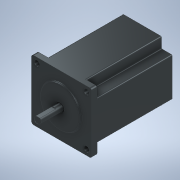
# Autodesk Inventor part: 0x002
Saved by Autodesk Inventor 2020 (Build 240168000, 168)
## iProperties
Created: 2024-01-28
Part Number: 0x002
Material: Iron, Cast
Document SubType Name: Modeling
Designer: Scott Bricker
Density: 7.15 g/cm^3
Appearance: Iron Gray
Mass: 1598.08 g
Surface Area: 245.33 cm^2
Volume: 223.508 cm^3
Project: Motorized Rotator Mount
Description: Stepper Motor
Engineer: Scott Bricker
Author: Scott Bricker
Title: Stepper Motor
Comments: Re-modeled replica of StepperOnline NEMA23 stepper motor for modeling purposes.
Revision Number: v1.0
Autodesk Inventor part; units mm, degrees
ref_plane "YZ Plane" through (0, 0, 0) normal (1, 0, 0) x (0, 1, 0)
ref_plane "XZ Plane" through (0, 0, 0) normal (0, 1, 0) x (-1, 0, 0)
ref_plane "XY Plane" through (0, 0, 0) normal (0, 0, 1) x (1, 0, 0)
sketch "Sketch1" plane through (0, 0, 0) normal (0, 0, 1) x (1, 0, 0)
  line L0 (11.16, 0) -> (46.14, 0)
  line L1 (57.3, 11.16) -> (57.3, 46.14)
  line L2 (46.14, 57.3) -> (11.16, 57.3)
  line L3 (0, 46.14) -> (0, 11.16)
  line L4 (0, 0) -> (0, 10.16)
  line L5 (1, 10.16) -> (9.16, 10.16)
  line L6 (10.16, 9.16) -> (10.16, 1)
  line L7 (57.3, 0) -> (47.14, 0)
  line L8 (47.14, 1) -> (47.14, 9.16)
  line L9 (48.14, 10.16) -> (56.3, 10.16)
  line L10 (47.14, 56.3) -> (47.14, 48.14)
  line L11 (48.14, 47.14) -> (56.3, 47.14)
  line L12 (10.16, 56.3) -> (10.16, 48.14)
  line L13 (1, 47.14) -> (9.16, 47.14)
  arc A0 (9.16, 47.14) -> (10.16, 48.14) centre (9.16, 48.14) ccw
  arc A1 (47.14, 48.14) -> (48.14, 47.14) centre (48.14, 48.14) ccw
  arc A2 (10.16, 9.16) -> (9.16, 10.16) centre (9.16, 9.16) ccw
  arc A3 (48.14, 10.16) -> (47.14, 9.16) centre (48.14, 9.16) ccw
  arc A4 (11.16, 57.3) -> (10.16, 56.3) centre (11.16, 56.3) ccw
  arc A5 (47.14, 56.3) -> (46.14, 57.3) centre (46.14, 56.3) ccw
  arc A6 (57.3, 46.14) -> (56.3, 47.14) centre (56.3, 46.14) ccw
  arc A7 (56.3, 10.16) -> (57.3, 11.16) centre (56.3, 11.16) ccw
  arc A8 (46.14, 0) -> (47.14, 1) centre (46.14, 1) ccw
  arc A9 (10.16, 1) -> (11.16, 0) centre (11.16, 1) ccw
  arc A10 (0, 11.16) -> (1, 10.16) centre (1, 11.16) ccw
  arc A11 (1, 47.14) -> (0, 46.14) centre (1, 46.14) ccw
  point P0 (57.3, 57.3)
  point P1 (0, 47.14)
  point P2 (10.16, 10.16)
  point P3 (47.14, 10.16)
  point P4 (47.14, 47.14)
  point P5 (10.16, 47.14)
  point P6 (10.16, 57.3)
  point P7 (47.14, 57.3)
  point P8 (57.3, 10.16)
  dimension "d25" = 57.3
  dimension "d26" = 57.3
  dimension "d27" = 10.16
  dimension "d28" = 10.16
  dimension "d29" = 10.16
  dimension "d30" = 10.16
  dimension "d31" = 1
  constraints: 31 point on line, 28 end point, 24 point on circle, 24 tangent, 12 centre point, 11 equal radius, 8 perpendicular, 1 horizontal
  measures "d25" distance of L4.start L7.start
  measures "d26" distance of L7.start point (57.3, 57.3)
  measures "d27" distance of L4.start L4.end
  measures "d28" distance of L4.end point (10.16, 10.16)
  measures "d29" distance of L7.start L7.end
  measures "d30" distance of point (47.14, 57.3) point (47.14, 47.14)
  measures "d31" radius of A0
extrude "Extrusion4" add sketch "Sketch1" along normal blind 76.5
sketch "Sketch4" plane through (0, 0, 76.5) normal (0, 0, 1) x (1, 0, 0)
  arc A0 (10.16, 1) -> (11.16, 0) centre (11.16, 1) ccw projected
  line L0 (11.16, 0) -> (46.14, 0) projected
  arc A1 (46.14, 0) -> (47.14, 1) centre (46.14, 1) ccw projected
  line L1 (47.14, 1) -> (47.14, 9.16) projected
  arc A2 (48.14, 10.16) -> (47.14, 9.16) centre (48.14, 9.16) ccw projected
  line L2 (48.14, 10.16) -> (56.3, 10.16) projected
  arc A3 (56.3, 10.16) -> (57.3, 11.16) centre (56.3, 11.16) ccw projected
  line L3 (57.3, 11.16) -> (57.3, 46.14) projected
  arc A4 (57.3, 46.14) -> (56.3, 47.14) centre (56.3, 46.14) ccw projected
  line L4 (56.3, 47.14) -> (48.14, 47.14) projected
  arc A5 (47.14, 48.14) -> (48.14, 47.14) centre (48.14, 48.14) ccw projected
  line L5 (47.14, 48.14) -> (47.14, 56.3) projected
  arc A6 (47.14, 56.3) -> (46.14, 57.3) centre (46.14, 56.3) ccw projected
  line L6 (46.14, 57.3) -> (11.16, 57.3) projected
  arc A7 (11.16, 57.3) -> (10.16, 56.3) centre (11.16, 56.3) ccw projected
  line L7 (10.16, 56.3) -> (10.16, 48.14) projected
  arc A8 (9.16, 47.14) -> (10.16, 48.14) centre (9.16, 48.14) ccw projected
  line L8 (9.16, 47.14) -> (1, 47.14) projected
  arc A9 (1, 47.14) -> (0, 46.14) centre (1, 46.14) ccw projected
  line L9 (0, 46.14) -> (0, 11.16) projected
  arc A10 (0, 11.16) -> (1, 10.16) centre (1, 11.16) ccw projected
  line L10 (1, 10.16) -> (9.16, 10.16) projected
  arc A11 (10.16, 9.16) -> (9.16, 10.16) centre (9.16, 9.16) ccw projected
  line L11 (10.16, 9.16) -> (10.16, 1) projected
  line L12 (0, 0) -> (57.3, 0)
  line L13 (57.3, 0) -> (57.3, 57.3)
  line L14 (57.3, 57.3) -> (0, 57.3)
  line L15 (0, 57.3) -> (0, 0)
  line L16 (0, 57.3) -> (5.08, 57.3)
  line L17 (5.08, 57.3) -> (5.08, 52.22)
  line L18 (57.3, 0) -> (52.22, 0)
  line L19 (52.22, 0) -> (52.22, 5.08)
  circle A12 centre (52.22, 52.22) radius 2.6
  circle A13 centre (5.08, 5.08) radius 2.6
  circle A14 centre (52.22, 5.08) radius 2.6
  circle A15 centre (5.08, 52.22) radius 2.6
  dimension "d34" = 5.08
  dimension "d35" = 5.08
  dimension "d36" = 5.08
  dimension "d37" = 5.08
  dimension "d38" = 5.2
  dimension "d39" = 5.2
  dimension "d40" = 5.2
  dimension "d41" = 5.2
  constraints: 16 end point, 4 centre point, 4 perpendicular, 2 coincident, 2 horizontal, 2 point on line
  measures "d34" distance of L14.end L16.end
  measures "d35" distance of L16.end L17.end
  measures "d36" distance of L12.end L18.end
  measures "d37" distance of L18.end L19.end
  measures "d38" diameter of A12
  measures "d39" diameter of A13
  measures "d40" diameter of A14
  measures "d41" diameter of A15
extrude "Extrusion5" add sketch "Sketch4" against normal blind 5
fillet "Fillet1" radius 2 4 edges at (57.3, 57.3, 74) (57.3, 0, 74) (0, 57.3, 74) (0, 0, 74)
sketch "Sketch5" plane through (0, 0, 76.5) normal (0, 0, 1) x (1, 0, 0)
  arc A0 (0, 2) -> (2, 0) centre (2, 2) ccw projected
  line L0 (2, 0) -> (55.3, 0) projected
  arc A1 (55.3, 0) -> (57.3, 2) centre (55.3, 2) ccw projected
  line L1 (57.3, 2) -> (57.3, 55.3) projected
  arc A2 (57.3, 55.3) -> (55.3, 57.3) centre (55.3, 55.3) ccw projected
  line L2 (55.3, 57.3) -> (2, 57.3) projected
  arc A3 (2, 57.3) -> (0, 55.3) centre (2, 55.3) ccw projected
  line L3 (0, 55.3) -> (0, 2) projected
  circle A4 centre (52.22, 52.22) radius 2.6 projected
  circle A5 centre (5.08, 52.22) radius 2.6 projected
  circle A6 centre (52.22, 5.08) radius 2.6 projected
  circle A7 centre (5.08, 5.08) radius 2.6 projected
  circle A8 centre (28.65, 28.65) radius 19.05
  point P0 (0, 0)
  dimension "d45" = 38.1
  constraints: 1 centre point
  measures "d45" diameter of A8
extrude "Extrusion6" add sketch "Sketch5" along normal blind 1.6 contours A8
sketch "Sketch6" plane through (28.65, 28.65, 78.1) normal (0, 0, 1) x (1, 0, 0)
  circle A0 centre (0, 0) radius 3.175
  point P0 (-28.65, -28.65)
  dimension "d48" = 6.35
  constraints: 1 centre point
  measures "d48" diameter of A0
extrude "Extrusion7" add sketch "Sketch6" along normal blind 6
sketch "Sketch7" plane through (28.65, 28.65, 84.1) normal (0, 0, 1) x (1, 0, 0)
  arc A0 (-1.9572, 2.5) -> (1.9572, 2.5) centre (0, 0) ccw
  circle A1 centre (0, 0) radius 3.175 projected
  line L0 (0, 0) -> (0, 2.5)
  line L1 (-1.9572, 2.5) -> (1.9572, 2.5)
  point P0 (-28.65, -28.65)
  dimension "d51" = 2.5
  constraints: 4 end point, 4 point on circle, 1 centre point, 1 horizontal, 1 vertical
  measures "d51" distance of L0.start L0.end
extrude "Extrusion8" add sketch "Sketch7" along normal blind 15 contours L1 A0
sketch "Sketch8" plane through (28.65, 28.65, 78.1) normal (0, 0, 1) x (1, 0, 0)
  circle A0 centre (0, 0) radius 3.175
  circle A1 centre (0, 0) radius 4
  point P0 (-28.65, -28.65)
  dimension "d54" = 8
  constraints: 2 centre point, 1 coincident
  measures "d54" diameter of A1
extrude "Extrusion9" cut sketch "Sketch8" against normal blind 2 contours A0 | A1
fillet "Fillet2" radius 0.5 2 edges at (9.6, 28.65, 78.1) (9.6, 28.65, 76.5)
body "Solid2"
